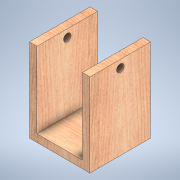
# Autodesk Inventor part: clutch02-forkBase
Saved by Autodesk Inventor 2021 (Build 250183000, 183)
## iProperties
Created: 2020-07-03
Part Number: clutch02-forkBase
Material: Wood (Birch)
Document SubType Name: Modeling
Designer: robst
Density: 0.55 g/cm^3
Appearance: Birch - Natural Polished
Author: robst
Autodesk Inventor part; units mm, degrees
ref_plane "YZ Plane" through (0, 0, 0) normal (1, 0, 0) x (0, 1, 0)
ref_plane "XZ Plane" through (0, 0, 0) normal (0, 1, 0) x (-1, 0, 0)
ref_plane "XY Plane" through (0, 0, 0) normal (0, 0, 1) x (1, 0, 0)
sketch "Sketch1" plane through (0, 0, 0) normal (0, 1, 0) x (-1, 0, 0)
  line L0 (101.6, 101.6) -> (-101.6, 101.6)
  line L1 (-101.6, 101.6) -> (-101.6, -101.6)
  line L2 (-101.6, -101.6) -> (101.6, -101.6)
  line L3 (101.6, -101.6) -> (101.6, 101.6)
  line L4 (101.6, 101.6) -> (-101.6, -101.6) construction
  line L5 (-101.6, 101.6) -> (101.6, -101.6) construction
  point P0 (0, 0)
  dimension "d0" = 203.2
  dimension "d1" = 203.2
  constraints: 12 end point, 2 midpoint, 2 parallel, 1 horizontal, 1 perpendicular
  measures "d0" distance of L0.start L0.end
  measures "d1" distance of L1.end L0.end
extrude "Extrusion1" add sketch "Sketch1" against normal blind 25.4
sketch "Sketch2" plane through (0, 0, 0) normal (0, 1, 0) x (1, 0, 0)
  line L0 (-101.6, -101.6) -> (-101.6, 101.6) projected
  line L1 (101.6, -101.6) -> (-101.6, -101.6) projected
  line L2 (-101.6, 101.6) -> (-76.2, 101.6)
  line L3 (-76.2, 101.6) -> (-76.2, -101.6)
  line L4 (-76.2, -101.6) -> (-101.6, -101.6)
  line L5 (-101.6, -101.6) -> (-101.6, 101.6)
  line L6 (101.6, 101.6) -> (101.6, -101.6) projected
  line L7 (101.6, 101.6) -> (76.2, 101.6)
  line L8 (76.2, 101.6) -> (76.2, -101.6)
  line L9 (76.2, -101.6) -> (101.6, -101.6)
  line L10 (101.6, -101.6) -> (101.6, 101.6)
  point P0 (0, 0)
  dimension "d4" = 25.4
  dimension "d5" = 25.4
  constraints: 16 end point, 4 parallel, 2 horizontal, 2 perpendicular, 2 point on line
  measures "d4" distance of L3.end L4.end
  measures "d5" distance of L9.end L8.end
extrude "Extrusion2" add sketch "Sketch2" along normal blind 254
sketch "Sketch3" plane through (-101.6, -25.4, -101.6) normal (-1, 0, 0) x (0, 0, 1)
  circle A0 centre (101.6, 254) radius 12.7
  line L0 (0, 279.4) -> (203.2, 279.4) projected
  point P0 (101.6, 25.4)
  dimension "d8" = 25.4
  dimension "d9" = 25.4
  constraints: 1 centre point
  measures "d8" distance from line of A0.centre L0
  measures "d9" diameter of A0
extrude "Extrusion4" cut sketch "Sketch3" against normal through all
body "Solid1"
